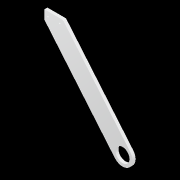
# Autodesk Inventor part: winch_support_starboard_aft
Saved by Autodesk Inventor 2020.2 (Build 242310000, 310)
## iProperties
Created: 2020-03-28
Part Number: winch_support_starboard_aft
Material: Aluminum 6061
Document SubType Name: Modeling
Designer: agmle
Density: 2.7 g/cm^3
Appearance: Aluminum - Flat
Mass: 170.379 g
Surface Area: 242.62 cm^2
Volume: 63.1034 cm^3
Author: agmle
Autodesk Inventor part; units mm, degrees
ref_plane "YZ Plane" through (0, 0, 0) normal (1, 0, 0) x (0, 1, 0)
ref_plane "XZ Plane" through (0, 0, 0) normal (0, 1, 0) x (-1, 0, 0)
ref_plane "XY Plane" through (0, 0, 0) normal (0, 0, 1) x (1, 0, 0)
sketch "Sketch1" plane through (0, 0, 0) normal (0, 0, 1) x (1, 0, 0)
  line L0 (-245.3259, 0) -> (63.2798, 244.4632) construction
  line L1 (63.2798, 244.4632) -> (245.3259, 0) construction
  line L2 (245.3259, 0) -> (-245.3259, 0) construction
  circle A0 centre (-245.3259, 0) radius 14.7955 construction
  circle A1 centre (245.3259, 0) radius 14.7955 construction
  arc A2 (-258.4559, 16.5751) -> (-232.1959, -16.5751) centre (-245.3259, 0) ccw construction
  arc A3 (229.0801, -13.5354) -> (261.5717, 13.5354) centre (245.3259, 0) ccw
  line L3 (-258.4559, 16.5751) -> (-47.8104, 183.4388) construction
  line L4 (-47.8104, 183.4388) -> (120.0143, 183.4388) construction
  line L5 (120.0143, 183.4388) -> (261.5717, 13.5354)
  line L6 (229.0801, -13.5354) -> (80.8402, 164.3888)
  line L7 (80.8402, 164.3888) -> (-3.7505, 164.3888) construction
  line L8 (-3.7505, 164.3888) -> (-232.1959, -16.5751) construction
  line L9 (120.0143, 183.4388) -> (80.8402, 183.4388)
  line L10 (80.8402, 183.4388) -> (80.8402, 164.3888)
  line L11 (63.2798, 244.4632) -> (63.2798, 173.9138) construction
  line L12 (63.2798, 173.9138) -> (112.8098, 173.9138) construction
  line L13 (112.8098, 173.9138) -> (121.7466, 181.3597) construction
  line L14 (88.0448, 173.9138) -> (79.1079, 166.4679) construction
  point P0 (0, 0)
  point P1 (0, 0)
  point P2 (80.8402, 173.9138)
  dimension "d0" = 304.8
  dimension "d1" = 393.7
  dimension "d2" = 490.6518
  dimension "d3" = 29.591
  dimension "d4" = 6.35
  dimension "d5" = 19.05
  dimension "d6" = 164.3888
  dimension "d34" = 24.765
  constraints: 30 end point, 6 coincident, 5 parallel, 4 centre point, 4 point on circle, 4 point on line, 4 tangent, 3 horizontal, 3 midpoint, 2 equal radius, 2 perpendicular, 2 vertical
  measures "d0" distance of L0.end L1.end
  measures "d1" distance of L0.start L0.end
  measures "d2" distance of L1.end L0.start
  measures "d3" diameter of A0
  measures "d4" radial gap between concentric circles of A0 A2
  measures "d5" distance between parallel lines of L7 L4
  measures "d6" distance between parallel lines of L2 L7
  measures "d34" distance of L12.end L14.start
extrude "Frame" add sketch "Sketch1" along normal blind 6.35
sketch "Sketch2" plane through (0, 0, 6.35) normal (0, 0, 1) x (1, 0, 0)
  arc A0 (229.0801, -13.5354) -> (261.5717, 13.5354) centre (245.3259, 0) ccw projected
  point P0 (0, 0)
  point P1 (245.3259, 0)
  constraints: 1 coincident
hole "Struts" at (245.3259, 0, 6.35) direction (0, 0, -1) diameter 29.591 end through all
fillet "Edge Break" radius 5 1 edges at (120.0143, 183.4388, 3.175)
sketch "Sketch3" plane through (0, 0, 0) normal (0, 0, -1) x (-1, 0, 0)
  line L0 (-261.5717, 13.5354) -> (-121.5136, 181.6393) construction
  line L1 (-121.751, 181.3544) -> (-112.8205, 173.9138) construction
  line L2 (-112.8205, 173.9138) -> (-88.0555, 173.9138) construction
  line L3 (-88.0555, 173.9138) -> (-79.125, 166.4732) construction
  line L4 (-80.8402, 164.3888) -> (-229.0801, -13.5354) construction
  line L5 (-261.5717, 13.5354) -> (-121.5136, 181.6393) construction
  line L6 (-80.8402, 183.4388) -> (-80.8402, 164.3888) construction
  point P0 (0, 0)
  point P1 (-80.8402, 173.9138)
  dimension "d33" = 24.765
  constraints: 6 end point, 2 perpendicular, 2 point on line, 1 coincident, 1 horizontal, 1 midpoint, 1 parallel
  measures "d33" distance of L2.end point (-112.821, 173.914)
hole "Mount Bolts" at (88.0555, 173.9138, 0) at (112.8205, 173.9138, 0) direction (0, 0, 1) diameter 3.4036 end through all countersink diameter 6.2992 countersink angle 90 clearance for "Flat Head Machine Screw" size "M3" standard "Ansi Metric M Profile"
body "Solid1"
